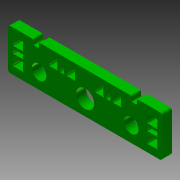
# Autodesk Inventor part: floor_sideA
Saved by Autodesk Inventor 2012 SP1 (Build 160190100, 190)
## iProperties
Created: 2011-10-14
Part Number: floor_sideA
Document SubType Name: Modeling
Designer: cramera
Density: 0.952 g/cm^3
Material: High Density Polyethylene
Mass: 82.2835 g
Surface Area: 326.179 cm^2
Volume: 86.4323 cm^3
Autodesk Inventor part; units mm, degrees
ref_plane "YZ Plane" through (0, 0, 0) normal (1, 0, 0) x (0, 1, 0)
ref_plane "XZ Plane" through (0, 0, 0) normal (0, 1, 0) x (-1, 0, 0)
ref_plane "XY Plane" through (0, 0, 0) normal (0, 0, 1) x (1, 0, 0)
derived "skeleton.ipt"
sketch "STOCK_12MM" plane through (0, 0, 0) normal (0, 0, 1) x (1, 0, 0)
  line L0 (457.2, 914.4) -> (457.2, 0)
  line L1 (0, 0) -> (457.2, 0)
  line L2 (457.2, 0) -> (457.2, 914.4)
  line L3 (457.2, 914.4) -> (0, 914.4)
  line L4 (0, 914.4) -> (0, 0)
  constraints: 10 end point
sketch "THROUGH-CUT" plane through (0, 0, 0) normal (0, 0, 1) x (1, 0, 0)
  line L0 (156.1543, 91.5886) -> (161.8241, 91.5886)
  arc A0 (161.8241, 91.5886) -> (164.0692, 93.8336) centre (162.9467, 92.7111) ccw
  line L1 (164.0692, 93.8336) -> (164.0692, 101.6625)
  arc A1 (164.0692, 101.6625) -> (161.8241, 103.9076) centre (162.9467, 102.785) ccw
  line L2 (161.8241, 103.9076) -> (156.1543, 103.9076)
  arc A2 (156.1543, 103.9076) -> (153.9092, 103.9076) centre (155.0317, 102.785) ccw
  arc A3 (153.9092, 103.9076) -> (153.9092, 101.6625) centre (155.0317, 102.785) ccw
  line L3 (153.9092, 101.6625) -> (153.9092, 93.8336)
  arc A4 (153.9092, 93.8336) -> (153.9092, 91.5886) centre (155.0317, 92.7111) ccw
  arc A5 (62.0974, 90.6996) -> (64.3424, 92.9446) centre (63.2199, 91.8221) ccw
  line L4 (64.3424, 92.9446) -> (64.3424, 98.6145)
  arc A6 (64.3424, 98.6145) -> (62.0974, 100.8596) centre (63.2199, 99.737) ccw
  line L5 (62.0974, 100.8596) -> (54.2685, 100.8596)
  arc A7 (54.2685, 100.8596) -> (52.0234, 100.8596) centre (53.146, 99.737) ccw
  arc A8 (52.0234, 100.8596) -> (52.0234, 98.6145) centre (53.146, 99.737) ccw
  line L6 (52.0234, 98.6145) -> (52.0234, 92.9446)
  arc A9 (52.0234, 92.9446) -> (54.2685, 90.6996) centre (53.146, 91.8221) ccw
  line L7 (54.2685, 90.6996) -> (62.0974, 90.6996)
  line L8 (230.6489, 71.1006) -> (230.6489, 76.7705)
  arc A10 (230.6489, 76.7705) -> (230.6489, 79.0156) centre (229.5264, 77.893) ccw
  arc A11 (230.6489, 79.0156) -> (228.4039, 79.0156) centre (229.5264, 77.893) ccw
  line L9 (228.4039, 79.0156) -> (220.575, 79.0156)
  arc A12 (220.575, 79.0156) -> (218.3299, 79.0156) centre (219.4525, 77.893) ccw
  arc A13 (218.3299, 79.0156) -> (218.3299, 76.7705) centre (219.4525, 77.893) ccw
  line L10 (218.3299, 76.7705) -> (218.3299, 71.1006)
  arc A14 (218.3299, 71.1006) -> (220.575, 68.8556) centre (219.4525, 69.9781) ccw
  line L11 (220.575, 68.8556) -> (228.4039, 68.8556)
  arc A15 (228.4039, 68.8556) -> (230.6489, 68.8556) centre (229.5264, 69.9781) ccw
  arc A16 (230.6489, 68.8556) -> (230.6489, 71.1006) centre (229.5264, 69.9781) ccw
  arc A17 (64.3424, 68.8556) -> (64.3424, 71.1006) centre (63.2199, 69.9781) ccw
  line L12 (64.3424, 71.1006) -> (64.3424, 76.7705)
  arc A18 (64.3424, 76.7705) -> (62.0974, 79.0156) centre (63.2199, 77.893) ccw
  line L13 (62.0974, 79.0156) -> (54.2685, 79.0156)
  arc A19 (54.2685, 79.0156) -> (52.0234, 79.0156) centre (53.146, 77.893) ccw
  arc A20 (52.0234, 79.0156) -> (52.0234, 76.7705) centre (53.146, 77.893) ccw
  line L14 (52.0234, 76.7705) -> (52.0234, 71.1006)
  arc A21 (52.0234, 71.1006) -> (52.0234, 68.8556) centre (53.146, 69.9781) ccw
  arc A22 (52.0234, 68.8556) -> (54.2685, 68.8556) centre (53.146, 69.9781) ccw
  line L15 (54.2685, 68.8556) -> (62.0974, 68.8556)
  arc A23 (62.0974, 68.8556) -> (64.3424, 68.8556) centre (63.2199, 69.9781) ccw
  line L16 (120.8483, 91.5886) -> (126.5181, 91.5886)
  arc A24 (126.5181, 91.5886) -> (128.7632, 91.5886) centre (127.6407, 92.7111) ccw
  arc A25 (128.7632, 91.5886) -> (128.7632, 93.8336) centre (127.6407, 92.7111) ccw
  line L17 (128.7632, 93.8336) -> (128.7632, 101.6625)
  arc A26 (128.7632, 101.6625) -> (126.5181, 103.9076) centre (127.6407, 102.785) ccw
  line L18 (126.5181, 103.9076) -> (120.8483, 103.9076)
  arc A27 (120.8483, 103.9076) -> (118.6032, 101.6625) centre (119.7257, 102.785) ccw
  line L19 (118.6032, 101.6625) -> (118.6032, 93.8336)
  arc A28 (118.6032, 93.8336) -> (118.6032, 91.5886) centre (119.7257, 92.7111) ccw
  arc A29 (118.6032, 91.5886) -> (120.8483, 91.5886) centre (119.7257, 92.7111) ccw
  arc A30 (167.3712, 93.8336) -> (169.6163, 91.5886) centre (168.4937, 92.7111) ccw
  line L20 (169.6163, 91.5886) -> (170.2061, 91.5886)
  arc A31 (170.2061, 91.5886) -> (172.4512, 93.8336) centre (171.3287, 92.7111) ccw
  line L21 (172.4512, 93.8336) -> (172.4512, 101.6625)
  arc A32 (172.4512, 101.6625) -> (170.2061, 103.9076) centre (171.3287, 102.785) ccw
  line L22 (170.2061, 103.9076) -> (169.6163, 103.9076)
  arc A33 (169.6163, 103.9076) -> (167.3712, 103.9076) centre (168.4937, 102.785) ccw
  arc A34 (167.3712, 103.9076) -> (167.3712, 101.6625) centre (168.4937, 102.785) ccw
  line L23 (167.3712, 101.6625) -> (167.3712, 93.8336)
  line L24 (230.6489, 84.5626) -> (230.6489, 85.1525)
  arc A35 (230.6489, 85.1525) -> (230.6489, 87.3976) centre (229.5264, 86.275) ccw
  arc A36 (230.6489, 87.3976) -> (228.4039, 87.3976) centre (229.5264, 86.275) ccw
  line L25 (228.4039, 87.3976) -> (220.575, 87.3976)
  arc A37 (220.575, 87.3976) -> (218.3299, 87.3976) centre (219.4525, 86.275) ccw
  arc A38 (218.3299, 87.3976) -> (218.3299, 85.1525) centre (219.4525, 86.275) ccw
  line L26 (218.3299, 85.1525) -> (218.3299, 84.5626)
  arc A39 (218.3299, 84.5626) -> (218.3299, 82.3176) centre (219.4525, 83.4401) ccw
  arc A40 (218.3299, 82.3176) -> (220.575, 82.3176) centre (219.4525, 83.4401) ccw
  line L27 (220.575, 82.3176) -> (228.4039, 82.3176)
  arc A41 (228.4039, 82.3176) -> (230.6489, 82.3176) centre (229.5264, 83.4401) ccw
  arc A42 (230.6489, 82.3176) -> (230.6489, 84.5626) centre (229.5264, 83.4401) ccw
  circle A43 centre (141.3362, 78.5076) radius 11.1125
  arc A44 (96.7592, 91.5886) -> (99.0043, 91.5886) centre (97.8817, 92.7111) ccw
  line L28 (99.0043, 91.5886) -> (104.6741, 91.5886)
  arc A45 (104.6741, 91.5886) -> (106.9192, 93.8336) centre (105.7967, 92.7111) ccw
  line L29 (106.9192, 93.8336) -> (106.9192, 101.6625)
  arc A46 (106.9192, 101.6625) -> (106.9192, 103.9076) centre (105.7967, 102.785) ccw
  arc A47 (106.9192, 103.9076) -> (104.6741, 103.9076) centre (105.7967, 102.785) ccw
  line L30 (104.6741, 103.9076) -> (99.0043, 103.9076)
  arc A48 (99.0043, 103.9076) -> (96.7592, 103.9076) centre (97.8817, 102.785) ccw
  arc A49 (96.7592, 103.9076) -> (96.7592, 101.6625) centre (97.8817, 102.785) ccw
  line L31 (96.7592, 101.6625) -> (96.7592, 93.8336)
  arc A50 (96.7592, 93.8336) -> (96.7592, 91.5886) centre (97.8817, 92.7111) ccw
  line L32 (64.3424, 84.5626) -> (64.3424, 85.1525)
  arc A51 (64.3424, 85.1525) -> (64.3424, 87.3976) centre (63.2199, 86.275) ccw
  arc A52 (64.3424, 87.3976) -> (62.0974, 87.3976) centre (63.2199, 86.275) ccw
  line L33 (62.0974, 87.3976) -> (54.2685, 87.3976)
  arc A53 (54.2685, 87.3976) -> (52.0234, 87.3976) centre (53.146, 86.275) ccw
  arc A54 (52.0234, 87.3976) -> (52.0234, 85.1525) centre (53.146, 86.275) ccw
  line L34 (52.0234, 85.1525) -> (52.0234, 84.5626)
  arc A55 (52.0234, 84.5626) -> (54.2685, 82.3176) centre (53.146, 83.4401) ccw
  line L35 (54.2685, 82.3176) -> (62.0974, 82.3176)
  arc A56 (62.0974, 82.3176) -> (64.3424, 82.3176) centre (63.2199, 83.4401) ccw
  arc A57 (64.3424, 82.3176) -> (64.3424, 84.5626) centre (63.2199, 83.4401) ccw
  arc A58 (228.4039, 90.6996) -> (230.6489, 92.9446) centre (229.5264, 91.8221) ccw
  line L36 (230.6489, 92.9446) -> (230.6489, 98.6145)
  arc A59 (230.6489, 98.6145) -> (228.4039, 100.8596) centre (229.5264, 99.737) ccw
  line L37 (228.4039, 100.8596) -> (220.575, 100.8596)
  arc A60 (220.575, 100.8596) -> (218.3299, 100.8596) centre (219.4525, 99.737) ccw
  arc A61 (218.3299, 100.8596) -> (218.3299, 98.6145) centre (219.4525, 99.737) ccw
  line L38 (218.3299, 98.6145) -> (218.3299, 92.9446)
  arc A62 (218.3299, 92.9446) -> (218.3299, 90.6996) centre (219.4525, 91.8221) ccw
  arc A63 (218.3299, 90.6996) -> (220.575, 90.6996) centre (219.4525, 91.8221) ccw
  line L39 (220.575, 90.6996) -> (228.4039, 90.6996)
  line L40 (112.4663, 91.5886) -> (113.0561, 91.5886)
  arc A64 (113.0561, 91.5886) -> (115.3012, 91.5886) centre (114.1787, 92.7111) ccw
  arc A65 (115.3012, 91.5886) -> (115.3012, 93.8336) centre (114.1787, 92.7111) ccw
  line L41 (115.3012, 93.8336) -> (115.3012, 101.6625)
  circle A66 centre (198.4862, 78.5076) radius 9.04
  circle A67 centre (84.1862, 78.5076) radius 9.04
  arc A68 (115.3012, 101.6625) -> (113.0561, 103.9076) centre (114.1787, 102.785) ccw
  line L42 (113.0561, 103.9076) -> (112.4663, 103.9076)
  arc A69 (112.4663, 103.9076) -> (110.2212, 103.9076) centre (111.3437, 102.785) ccw
  arc A70 (110.2212, 103.9076) -> (110.2212, 101.6625) centre (111.3437, 102.785) ccw
  line L43 (110.2212, 101.6625) -> (110.2212, 93.8336)
  arc A71 (110.2212, 93.8336) -> (110.2212, 91.5886) centre (111.3437, 92.7111) ccw
  arc A72 (110.2212, 91.5886) -> (112.4663, 91.5886) centre (111.3437, 92.7111) ccw
  arc A73 (153.9092, 91.5886) -> (156.1543, 91.5886) centre (155.0317, 92.7111) ccw
  line L44 (177.9983, 91.5886) -> (183.6681, 91.5886)
  arc A74 (183.6681, 91.5886) -> (185.9132, 91.5886) centre (184.7907, 92.7111) ccw
  arc A75 (185.9132, 91.5886) -> (185.9132, 93.8336) centre (184.7907, 92.7111) ccw
  line L45 (185.9132, 93.8336) -> (185.9132, 101.6625)
  arc A76 (185.9132, 101.6625) -> (183.6681, 103.9076) centre (184.7907, 102.785) ccw
  line L46 (183.6681, 103.9076) -> (177.9983, 103.9076)
  arc A77 (177.9983, 103.9076) -> (175.7532, 103.9076) centre (176.8757, 102.785) ccw
  arc A78 (175.7532, 103.9076) -> (175.7532, 101.6625) centre (176.8757, 102.785) ccw
  line L47 (175.7532, 101.6625) -> (175.7532, 93.8336)
  arc A79 (175.7532, 93.8336) -> (175.7532, 91.5886) centre (176.8757, 92.7111) ccw
  arc A80 (175.7532, 91.5886) -> (177.9983, 91.5886) centre (176.8757, 92.7111) ccw
  line L48 (197.0257, 110.2576) -> (85.6467, 110.2576)
  arc A81 (85.6467, 110.2576) -> (84.0592, 108.6701) centre (85.6467, 108.6701) ccw
  line L49 (84.0592, 108.6701) -> (84.0574, 105.4951)
  arc A82 (82.4699, 103.9076) -> (84.0574, 105.4951) centre (82.4699, 105.4951) ccw
  line L50 (82.4699, 103.9076) -> (78.6299, 103.9076)
  arc A83 (77.0424, 105.4951) -> (78.6299, 103.9076) centre (78.6299, 105.4951) ccw
  line L51 (77.0424, 105.4951) -> (77.0424, 108.6701)
  arc A84 (77.0424, 108.6701) -> (75.4549, 110.2576) centre (75.4549, 108.6701) ccw
  line L52 (75.4549, 110.2576) -> (48.8484, 110.2576)
  arc A85 (48.8484, 110.2576) -> (45.6734, 107.0826) centre (48.8484, 107.0826) ccw
  line L53 (45.6734, 107.0826) -> (45.6734, 62.6326)
  arc A86 (45.6734, 62.6326) -> (48.8484, 59.4576) centre (48.8484, 62.6326) ccw
  line L54 (48.8484, 59.4576) -> (233.8239, 59.4576)
  arc A87 (233.8239, 59.4576) -> (236.9989, 62.6326) centre (233.8239, 62.6326) ccw
  line L55 (236.9989, 62.6326) -> (236.9989, 107.0826)
  arc A88 (236.9989, 107.0826) -> (233.8239, 110.2576) centre (233.8239, 107.0826) ccw
  line L56 (233.8239, 110.2576) -> (207.2174, 110.2576)
  arc A89 (207.2174, 110.2576) -> (205.6299, 108.6701) centre (207.2174, 108.6701) ccw
  line L57 (205.6299, 108.6701) -> (205.6299, 105.4951)
  arc A90 (204.0424, 103.9076) -> (205.6299, 105.4951) centre (204.0424, 105.4951) ccw
  line L58 (204.0424, 103.9076) -> (200.2024, 103.9076)
  arc A91 (198.6149, 105.4951) -> (200.2024, 103.9076) centre (200.2024, 105.4951) ccw
  line L59 (198.6149, 105.4951) -> (198.6132, 108.6701)
  arc A92 (198.6132, 108.6701) -> (197.0257, 110.2576) centre (197.0257, 108.6701) ccw
  dimension "d5" = 18.08
  dimension "d6" = 18.08
  dimension "d7" = 114.3
  dimension "d8" = 22.225
  constraints: 180 point on circle, 120 end point, 93 centre point
  measures "d5" diameter of A67
  measures "d6" diameter of A66
  measures "d7" distance of A66.centre A67.centre
  measures "d8" diameter of A43
extrude "Extrusion1" add sketch "THROUGH-CUT" along normal blind 12
equation "\"d6\" = d5"
equation "\"d1\" = StockThickness"
equation "\"StockThickness\" = 12"
body "Solid1"
